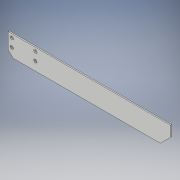
# Autodesk Inventor part: SideBracket
Saved by Autodesk Inventor 2019.3 (Build 233278000, 278)
## iProperties
Created: 2019-01-26
Part Number: SideBracket
Material: Generic
Document SubType Name: Modeling
Designer: mark
Density: 1 g/cm^3
Appearance: Default
Author: mark
Autodesk Inventor part; units mm, degrees
ref_plane "YZ Plane" through (0, 0, 0) normal (1, 0, 0) x (0, 1, 0)
ref_plane "XZ Plane" through (0, 0, 0) normal (0, 1, 0) x (-1, 0, 0)
ref_plane "XY Plane" through (0, 0, 0) normal (0, 0, 1) x (1, 0, 0)
sketch "Sketch1" plane through (0, 0, 0) normal (0, 0, 1) x (1, 0, 0)
  line L0 (0, 0) -> (400, 0)
  line L1 (400, 0) -> (400, -25.375)
  line L2 (0, -38.2) -> (12.55, -50.75)
  line L3 (400, -25.375) -> (374.625, -50.75)
  line L4 (0, -38.2) -> (0, 0)
  line L5 (374.625, -50.75) -> (12.55, -50.75)
  circle A0 centre (9, -9) radius 4
  circle A1 centre (9, -29.2) radius 4
  circle A2 centre (67.2, -9) radius 4
  circle A3 centre (67.2, -29.2) radius 4
  dimension "d3" = 8
  dimension "d4" = 8
  dimension "d5" = 8
  dimension "d6" = 8
  dimension "d10" = 9
  dimension "d11" = 9
  dimension "d12" = 9
  dimension "d13" = 9
  dimension "d15" = 20.2
  dimension "d16" = 58.2
  dimension "d18" = 12.55
  dimension "d19" = 400
  dimension "d20" = 50.75
  dimension "d21" = 25.375
  dimension "d22" = 20.2
  dimension "d23" = 58.2
  dimension "d24" = 12.55
  dimension "d25" = 25.375
  constraints: 12 end point, 4 centre point, 3 perpendicular, 1 coincident, 1 horizontal
  measures "d3" diameter of A0
  measures "d4" diameter of A1
  measures "d5" diameter of A2
  measures "d6" diameter of A3
  measures "d10" distance from line of L0 A2.centre
  measures "d11" distance from line of L0 A0.centre
  measures "d12" distance from line of L4 A0.centre
  measures "d13" distance from line of L4 A1.centre
  measures "d15" distance of A2.centre A3.centre
  measures "d16" distance of A1.centre A3.centre
  measures "d18" horizontal distance of L2.start L2.end
  measures "d19" distance of L0.end point (0, 0)
  measures "d20" distance between parallel lines of L5 L0
  measures "d21" distance from line of L5 L1.end
  measures "d22" distance of A0.centre A1.centre
  measures "d23" distance of A0.centre A2.centre
  measures "d24" distance from line of L2.end L4
  measures "d25" horizontal distance of L3.end L1.end
extrude "Extrusion1" add sketch "Sketch1" along normal blind 3.1
body "Solid1"
